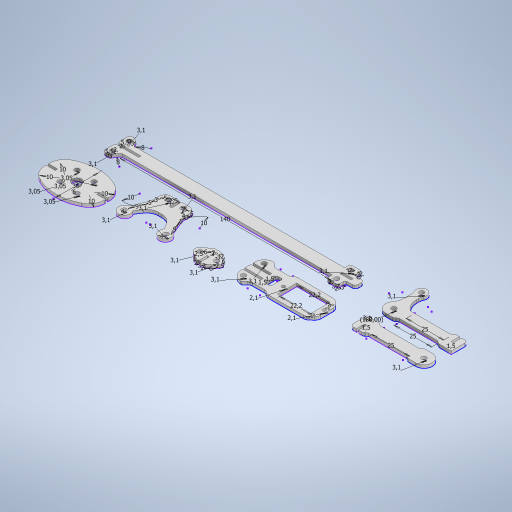
# Autodesk Inventor part: carbon_body_parts
Saved by Autodesk Inventor 2024 (Build 280153000, 153)
## iProperties
Created: 2024-04-09
Part Number: carbon_body_parts
Material: Generic
Document SubType Name: Modeling
Designer: nikop
Density: 1 g/cm^3
Appearance: Default
Author: nikop
Autodesk Inventor part; units mm, degrees
ref_plane "YZ Plane" through (0, 0, 0) normal (1, 0, 0) x (0, 1, 0)
ref_plane "XZ Plane" through (0, 0, 0) normal (0, 1, 0) x (-1, 0, 0)
ref_plane "XY Plane" through (0, 0, 0) normal (0, 0, 1) x (1, 0, 0)
sketch "Sketch1" plane through (0, 0, 0) normal (0, 1, 0) x (-1, 0, 0)
  circle A0 centre (58.9757, 25.2531) radius 1.525
  circle A1 centre (70.2894, 36.5668) radius 1.525
  circle A2 centre (57.915, 37.6275) radius 1.525
  circle A3 centre (71.3501, 24.1924) radius 1.525
  arc A4 (78.4011, 20.0636) -> (84.4011, 29.4099) centre (74.4027, 29.2295) ccw
  arc A5 (44.864, 29.4099) -> (50.864, 20.0636) centre (54.8624, 29.2295) ccw
  arc A6 (50.864, 20.0636) -> (78.4011, 20.0636) centre (64.6326, 46.7175) ccw
  arc A7 (84.4011, 32.4099) -> (78.4011, 41.7562) centre (74.4027, 32.5904) ccw
  arc A8 (50.864, 41.7562) -> (44.864, 32.4099) centre (54.8624, 32.5904) ccw
  arc A9 (78.4011, 41.7562) -> (50.864, 41.7562) centre (64.6326, 15.1024) ccw
  circle A10 centre (64.6326, 30.9099) radius 3
  line L0 (84.4011, 29.9099) -> (84.4011, 29.4099)
  line L1 (84.4011, 31.9099) -> (84.4011, 32.4099)
  line L2 (44.864, 29.9099) -> (44.864, 29.4099)
  line L3 (44.864, 31.9099) -> (44.864, 32.4099)
  line L4 (50.864, 31.6544) -> (50.864, 30.1544)
  line L5 (78.4011, 31.6599) -> (78.4011, 30.1599)
  line L6 (50.864, 30.1544) -> (50.864, 30.2794)
  line L7 (44.864, 29.9099) -> (44.864, 30.0349)
  line L8 (44.864, 31.7849) -> (44.864, 31.9099)
  line L9 (78.4011, 30.1599) -> (78.4011, 30.2849)
  line L10 (78.4011, 31.6599) -> (78.4011, 31.5349)
  line L11 (84.4011, 30.0349) -> (84.4011, 29.9099)
  line L12 (78.4011, 30.1599) -> (84.4011, 30.1599)
  line L13 (84.4011, 30.1599) -> (84.4011, 30.0349)
  line L14 (84.4011, 31.7849) -> (84.4011, 31.9099)
  line L15 (50.864, 30.1544) -> (44.864, 30.1544)
  line L16 (44.864, 30.1544) -> (44.864, 30.0349)
  line L17 (50.864, 31.6544) -> (44.864, 31.6544)
  line L18 (44.864, 31.6544) -> (44.864, 31.7849)
  line L19 (78.4011, 31.6599) -> (84.4011, 31.6599)
  line L20 (84.4011, 31.6599) -> (84.4011, 31.7849)
  line L21 (-81.7792, -0.1869) -> (-81.7792, -0.3869)
  arc A11 (-82.7792, -1.3869) -> (-81.7792, -0.3869) centre (-82.7792, -0.3869) ccw
  line L22 (-82.7792, -1.3869) -> (-86.2983, -1.3869)
  arc A12 (-86.2983, -1.3869) -> (-88.2983, -3.3869) centre (-86.2983, -3.3869) ccw
  line L23 (-88.2983, -3.3869) -> (-88.2983, -5.3869)
  arc A13 (-88.2983, -5.3869) -> (-86.2983, -7.3869) centre (-86.2983, -5.3869) ccw
  line L24 (-86.2983, -7.3869) -> (-82.7792, -7.3869)
  arc A14 (-81.7617, -8.3867) -> (-82.7792, -7.3869) centre (-82.7617, -8.3867) ccw
  line L25 (-81.7617, -8.3867) -> (-81.7617, -8.5869)
  line L26 (70.7017, -7.8869) -> (70.9617, -7.8869) construction
  line L27 (73.6839, -6.8202) -> (73.6839, -12.3202)
  arc A15 (71.1839, -13.3202) -> (73.6839, -12.3202) centre (71.4382, -10.331) ccw
  arc A16 (68.6839, -12.3202) -> (71.1839, -13.3202) centre (70.9296, -10.331) ccw
  line L28 (73.6995, -1.853) -> (73.6995, 3.647)
  arc A17 (73.6995, 3.647) -> (71.1995, 4.647) centre (71.4538, 1.6578) ccw
  arc A18 (71.1995, 4.647) -> (68.6839, 3.6292) centre (70.9452, 1.6578) ccw
  line L29 (-74.2088, -0.2378) -> (65.7912, -0.2378)
  line L30 (-74.2182, -8.5205) -> (65.7818, -8.5205)
  circle A19 centre (70.7017, 1.1131) radius 1.55
  circle A20 centre (70.7017, -9.8869) radius 1.55
  arc A21 (68.6839, -12.3202) -> (65.7818, -8.5205) centre (61.1656, -15.0543) ccw
  arc A22 (65.7912, -0.2378) -> (68.6839, 3.6292) centre (61.1303, 6.2643) ccw
  circle A23 centre (-77.7909, 0.3631) radius 1.55
  circle A24 centre (-77.7986, -9.1369) radius 1.55
  line L31 (-81.7617, -8.5869) -> (-81.7617, -11.5869)
  arc A25 (-81.7617, -11.5869) -> (-79.9139, -12.3522) centre (-80.175, -10.3693) ccw
  line L32 (-74.2182, -8.5205) -> (-74.2182, -11.5869)
  arc A26 (-76.0659, -12.3522) -> (-74.2182, -11.5869) centre (-75.8049, -10.3693) ccw
  line L33 (-79.9139, -12.3522) -> (-76.0659, -12.3522)
  line L34 (-81.7792, -0.1869) -> (-81.7792, 2.8131)
  line L35 (-74.2088, -0.2378) -> (-74.2088, 2.8131)
  arc A27 (-74.2088, 2.8131) -> (-76.0566, 3.5785) centre (-75.7955, 1.5956) ccw
  arc A28 (-79.9314, 3.5785) -> (-81.7792, 2.8131) centre (-80.1925, 1.5956) ccw
  line L36 (-79.9314, 3.5785) -> (-76.0566, 3.5785)
  line L37 (58.2017, -5.1369) -> (72.9149, -5.1369)
  line L38 (58.2017, -3.6369) -> (72.9149, -3.6369)
  line L39 (58.2017, -3.6369) -> (58.2017, -5.1369)
  arc A29 (72.9149, -3.6369) -> (73.6995, -1.853) centre (71.7084, -2.0417) ccw
  arc A30 (73.6839, -6.8202) -> (72.9149, -5.1369) centre (71.6866, -6.7153) ccw
  line L40 (-83.2983, -5.1369) -> (-75.7983, -5.1369)
  line L41 (-83.2983, -3.6369) -> (-75.7983, -3.6369)
  line L42 (-75.7983, -3.6369) -> (-75.7983, -5.1369)
  line L43 (-83.2983, -3.6369) -> (-83.2983, -5.1369)
  line L44 (-23.6125, 23.696) -> (-22.1233, 23.696)
  line L45 (-22.1233, 23.696) -> (-20.6203, 23.6923)
  arc A31 (-18.7385, 36.0083) -> (-20.6179, 36.6923) centre (-20.6455, 33.6924) ccw
  arc A32 (-20.6203, 23.6923) -> (-18.7409, 24.3763) centre (-20.648, 26.6922) ccw
  arc A33 (-23.634, 36.696) -> (-25.5134, 36.012) centre (-23.6063, 33.6962) ccw
  arc A34 (-25.4919, 24.3801) -> (-23.6125, 23.696) centre (-23.5848, 26.6959) ccw
  circle A35 centre (-27.6234, 30.215) radius 1.55
  circle A36 centre (-16.6231, 30.2237) radius 1.55
  line L46 (-25.5134, 36.012) -> (-30.1097, 32.1553)
  line L47 (-25.4919, 24.3801) -> (-30.0881, 28.2368)
  arc A37 (-30.1097, 32.1553) -> (-30.0881, 28.2368) centre (-28.5461, 30.2046) ccw
  line L48 (-18.7409, 24.3763) -> (-14.1446, 28.2331)
  line L49 (-18.7385, 36.0083) -> (-14.1422, 32.1515)
  arc A38 (-14.1446, 28.2331) -> (-14.1422, 32.1515) centre (-15.6963, 30.1933) ccw
  line L50 (-23.634, 36.696) -> (-23.1232, 36.696)
  line L51 (-21.1071, 36.6935) -> (-20.6179, 36.6923)
  line L52 (-22.8732, 30.1867) -> (-22.8732, 36.696)
  line L53 (-22.8732, 36.696) -> (-23.1232, 36.696)
  line L54 (-21.3733, 30.1867) -> (-21.3733, 36.6935)
  line L55 (-21.3733, 36.6935) -> (-21.1071, 36.6935)
  line L56 (-22.8732, 30.1867) -> (-21.3733, 30.1867)
  arc A39 (-117.1771, -18.2977) -> (-116.557, -15.6154) centre (-122.5569, -15.641) ccw
  arc A40 (-117.1771, -18.2977) -> (-110.9285, -18.2954) centre (-114.0522, -19.8741) ccw
  arc A41 (-111.557, -15.622) -> (-110.9285, -18.2954) centre (-105.557, -15.622) ccw
  arc A42 (-109.6182, -4.6979) -> (-111.557, -10.5979) centre (-101.6102, -10.5979) ccw
  arc A43 (-109.6182, -4.6979) -> (-114.0537, 4.0542) centre (-114.0537, -1.4458) ccw
  line L57 (-114.0537, 4.0542) -> (-118.7253, 4.0542)
  arc A44 (-118.7253, 4.0542) -> (-120.1395, 3.4684) centre (-118.7253, 2.0542) ccw
  line L58 (-120.1395, 3.4684) -> (-120.4679, 3.14)
  arc A45 (-121.8822, 2.5542) -> (-120.4679, 3.14) centre (-121.8822, 4.5542) ccw
  line L59 (-146.8822, 2.5542) -> (-148.5338, 3.5078)
  arc A46 (-148.5338, 3.5078) -> (-149.9966, 4.0093) centre (-149.8634, 2.0137) ccw
  line L60 (-149.9966, 4.0093) -> (-155.6682, 4.0093)
  arc A47 (-149.9966, -6.9907) -> (-148.5824, -6.4049) centre (-149.9966, -4.9907) ccw
  line L61 (-148.5824, -6.4049) -> (-148.254, -6.0765)
  arc A48 (-146.8822, -5.4458) -> (-148.254, -6.0765) centre (-146.7944, -7.4439) ccw
  arc A49 (-120.4679, -6.0316) -> (-121.8822, -5.4458) centre (-121.8822, -7.4458) ccw
  line L62 (-120.4679, -6.0316) -> (-119.4827, -7.0169)
  arc A50 (-116.557, -14.0847) -> (-119.4827, -7.0169) centre (-126.557, -14.0847) ccw
  arc A51 (-146.2322, 21.7443) -> (-144.8179, 21.1585) centre (-144.8179, 23.1585) ccw
  line L63 (-146.2322, 21.7443) -> (-146.5606, 22.0727)
  arc A52 (-146.5606, 22.0727) -> (-147.9748, 22.6585) centre (-147.9748, 20.6585) ccw
  line L64 (-147.9748, 22.6585) -> (-152.6464, 22.6585)
  arc A53 (-152.6464, 22.6585) -> (-158.1464, 17.1585) centre (-152.6464, 17.1585) ccw
  arc A54 (-158.1464, 17.1585) -> (-152.6464, 11.6585) centre (-152.6464, 17.1585) ccw
  line L65 (-152.6464, 11.6585) -> (-147.9748, 11.6585)
  arc A55 (-147.9748, 11.6585) -> (-146.5606, 12.2443) centre (-147.9748, 13.6585) ccw
  line L66 (-146.5606, 12.2443) -> (-146.2322, 12.5727)
  arc A56 (-144.8179, 13.1585) -> (-146.2322, 12.5727) centre (-144.8179, 11.1585) ccw
  arc A57 (-118.6935, 12.6308) -> (-119.8179, 13.1585) centre (-120.0634, 11.1736) ccw
  line L67 (-118.6935, 12.6308) -> (-118.3651, 12.3024)
  arc A58 (-118.3651, 12.3024) -> (-116.9509, 11.7166) centre (-116.9509, 13.7166) ccw
  line L68 (-116.9509, 11.7166) -> (-111.2793, 11.7166)
  arc A59 (-116.9509, 22.7166) -> (-118.3651, 22.1308) centre (-116.9509, 20.7166) ccw
  line L69 (-118.3651, 22.1308) -> (-118.6935, 21.8024)
  arc A60 (-119.8179, 21.1585) -> (-118.6935, 21.8024) centre (-120.196, 23.1224) ccw
  line L70 (-157.6682, -1.4907) -> (-157.6682, -4.9907)
  line L71 (-157.6682, -1.4907) -> (-157.6682, 2.0093)
  arc A61 (-157.6682, -4.9907) -> (-155.6682, -6.9907) centre (-155.6682, -4.9907) ccw
  line L72 (-109.2793, 17.2166) -> (-109.2793, 20.7166)
  line L73 (-109.2793, 17.2166) -> (-109.2793, 13.7166)
  arc A62 (-109.2793, 20.7166) -> (-111.2793, 22.7166) centre (-111.2793, 20.7166) ccw
  line L74 (-149.9966, -6.9907) -> (-151.1682, -6.9907)
  line L75 (-154.1651, -6.9907) -> (-155.6682, -6.9907)
  circle A63 centre (-114.0537, -1.4458) radius 1.55
  circle A64 centre (-114.0602, -19.8581) radius 1.55
  circle A65 centre (-152.6464, 17.1585) radius 1.55
  line L76 (-111.2793, 22.7166) -> (-112.7793, 22.7166)
  line L77 (-115.7793, 22.7166) -> (-116.9509, 22.7166)
  line L78 (-111.557, -15.622) -> (-111.557, -10.5979)
  line L79 (-116.557, -15.6154) -> (-116.557, -14.0847)
  line L80 (-121.8822, -5.4458) -> (-146.8822, -5.4458)
  line L81 (-121.8822, 2.5542) -> (-146.8822, 2.5542)
  line L82 (-144.8179, 13.1585) -> (-119.8179, 13.1585)
  line L83 (-144.8179, 21.1585) -> (-119.8179, 21.1585)
  line L84 (-155.6682, 4.0093) -> (-157.6682, 4.0093)
  line L85 (-157.6682, 4.0093) -> (-157.6682, 2.0093)
  line L86 (-111.2793, 11.7166) -> (-109.2793, 11.7166)
  line L87 (-111.2793, 11.7166) -> (-113.2793, 11.7166) construction
  line L88 (-109.2793, 11.7166) -> (-109.2793, 13.7166)
  line L89 (-151.2682, -6.9907) -> (-151.1682, -6.9907)
  line L90 (-154.0682, -6.9907) -> (-154.1651, -6.9907)
  line L91 (-115.6793, 22.7166) -> (-115.7793, 22.7166)
  line L92 (-112.8793, 22.7166) -> (-112.7793, 22.7166)
  line L93 (-151.6682, -6.9907) -> (-151.2682, -6.9907)
  line L94 (-153.6682, -1.4907) -> (-153.6682, -6.9907)
  line L95 (-153.6682, -6.9907) -> (-154.0682, -6.9907)
  line L96 (-113.2793, 17.2166) -> (-113.2793, 22.7166)
  line L97 (-113.2793, 22.7166) -> (-112.8793, 22.7166)
  line L98 (-115.2793, 22.7166) -> (-115.6793, 22.7166)
  line L99 (-113.2793, 17.2166) -> (-114.7793, 17.2166)
  line L100 (-114.7793, 17.2166) -> (-114.7793, 22.7166)
  line L101 (-114.7793, 22.7166) -> (-115.2793, 22.7166)
  line L102 (-153.6682, -1.4907) -> (-152.1682, -1.4907)
  line L103 (-152.1682, -1.4907) -> (-152.1682, -6.9907)
  line L104 (-152.1682, -6.9907) -> (-151.6682, -6.9907)
  line L105 (-47.726, 11.8652) -> (-47.014, 11.8652)
  arc A66 (-47.014, 11.8652) -> (-41.014, 17.8652) centre (-47.014, 17.8652) ccw
  arc A67 (-41.014, 27.5152) -> (-47.014, 33.5152) centre (-47.014, 27.5152) ccw
  line L106 (-47.014, 33.5152) -> (-47.726, 33.5152)
  line L107 (-89.264, 28.1152) -> (-89.264, 22.6902)
  line L108 (-89.264, 22.6902) -> (-89.264, 17.2652)
  line L109 (-47.726, 11.8652) -> (-49.6723, 13.8116)
  line L110 (-87.6912, 12.8652) -> (-64.2306, 12.8652)
  line L111 (-62.1093, 13.7439) -> (-62.0417, 13.8116)
  line L112 (-53.226, 14.6902) -> (-51.7936, 14.6902)
  line L113 (-53.226, 14.6902) -> (-59.9203, 14.6902)
  line L114 (-93.564, 22.6902) -> (-93.564, 18.6074)
  line L115 (-92.2884, 15.6787) -> (-90.4156, 13.9365)
  arc A68 (-93.564, 18.6074) -> (-92.2884, 15.6787) centre (-89.564, 18.6074) ccw
  arc A69 (-90.4156, 13.9365) -> (-87.6912, 12.8652) centre (-87.6912, 16.8652) ccw
  arc A70 (-49.6723, 13.8116) -> (-51.7936, 14.6902) centre (-51.7936, 11.6902) ccw
  arc A71 (-59.9203, 14.6902) -> (-62.0417, 13.8116) centre (-59.9203, 11.6902) ccw
  arc A72 (-64.2306, 12.8652) -> (-62.1093, 13.7439) centre (-64.2306, 15.8652) ccw
  line L116 (-47.726, 33.5152) -> (-49.6723, 31.5689)
  line L117 (-87.6912, 32.5152) -> (-64.2306, 32.5152)
  line L118 (-62.1093, 31.6366) -> (-62.0417, 31.5689)
  line L119 (-53.226, 30.6902) -> (-51.7936, 30.6902)
  line L120 (-53.226, 30.6902) -> (-59.9203, 30.6902)
  line L121 (-93.564, 22.6902) -> (-93.564, 26.7731)
  line L122 (-92.2884, 29.7018) -> (-90.4156, 31.444)
  arc A73 (-92.2884, 29.7018) -> (-93.564, 26.7731) centre (-89.564, 26.7731) ccw
  arc A74 (-87.6912, 32.5152) -> (-90.4156, 31.444) centre (-87.6912, 28.5152) ccw
  arc A75 (-51.7936, 30.6902) -> (-49.6723, 31.5689) centre (-51.7936, 33.6902) ccw
  arc A76 (-62.0417, 31.5689) -> (-59.9203, 30.6902) centre (-59.9203, 33.6902) ccw
  arc A77 (-62.1093, 31.6366) -> (-64.2306, 32.5152) centre (-64.2306, 29.5152) ccw
  line L123 (-57.226, 18.6902) -> (-59.164, 18.6902)
  line L124 (-60.164, 19.6902) -> (-60.164, 25.6902)
  line L125 (-56.226, 19.6902) -> (-56.226, 25.6902)
  line L126 (-57.226, 26.6902) -> (-59.164, 26.6902)
  arc A78 (-57.226, 18.6902) -> (-56.226, 19.6902) centre (-57.226, 19.6902) ccw
  arc A79 (-60.164, 19.6902) -> (-59.164, 18.6902) centre (-59.164, 19.6902) ccw
  arc A80 (-59.164, 26.6902) -> (-60.164, 25.6902) centre (-59.164, 25.6902) ccw
  arc A81 (-56.226, 25.6902) -> (-57.226, 26.6902) centre (-57.226, 25.6902) ccw
  line L127 (-41.014, 17.8652) -> (-41.014, 18.1902)
  line L128 (-89.264, 17.2652) -> (-89.264, 16.2652)
  line L129 (-89.264, 28.1152) -> (-89.264, 29.1152)
  line L130 (-89.264, 16.2652) -> (-67.064, 16.2652)
  line L131 (-89.264, 29.1152) -> (-67.064, 29.1152)
  line L132 (-67.064, 16.2652) -> (-67.064, 29.1152)
  line L133 (-41.014, 27.5152) -> (-41.014, 27.1902)
  line L134 (-41.014, 21.1902) -> (-41.014, 24.1902)
  circle A82 centre (-44.926, 29.5902) radius 1.55
  circle A83 centre (-44.926, 15.7902) radius 1.55
  circle A84 centre (-64.614, 22.6902) radius 1.05
  circle A85 centre (-91.714, 22.6902) radius 1.05
  line L135 (-41.014, 18.6902) -> (-41.014, 18.1902)
  line L136 (-53.226, 20.6902) -> (-41.014, 20.6902)
  line L137 (-41.014, 20.6902) -> (-41.014, 21.1902)
  line L138 (-53.226, 24.6902) -> (-41.014, 24.6902)
  line L139 (-41.014, 24.6902) -> (-41.014, 24.1902)
  line L140 (-41.014, 26.6902) -> (-41.014, 27.1902)
  line L141 (-53.226, 24.6902) -> (-53.226, 26.1902)
  line L142 (-53.226, 26.1902) -> (-41.014, 26.1902)
  line L143 (-41.014, 26.1902) -> (-41.014, 26.6902)
  line L144 (-53.226, 20.6902) -> (-53.226, 19.1902)
  line L145 (-53.226, 19.1902) -> (-41.014, 19.1902)
  line L146 (-41.014, 19.1902) -> (-41.014, 18.6902)
  line L147 (10.9194, 25.0056) -> (8.2063, 29.0278)
  line L148 (26.5678, 25.0056) -> (29.2808, 29.0278)
  line L149 (18.7436, 21.4792) -> (17.5517, 21.4792)
  line L150 (18.7436, 21.4792) -> (19.9355, 21.4792)
  arc A86 (10.9194, 25.0056) -> (17.5517, 21.4792) centre (17.5517, 29.4792) ccw
  arc A87 (19.9355, 21.4792) -> (26.5678, 25.0056) centre (19.9355, 29.4792) ccw
  circle A88 centre (4.7436, 31.4792) radius 1.55
  circle A89 centre (32.7436, 31.4792) radius 1.55
  circle A90 centre (13.9936, 10.9792) radius 1.55
  circle A91 centre (23.4936, 10.9792) radius 1.55
  line L151 (17.2436, 7.9792) -> (12.2436, 7.9792)
  arc A92 (8.708, 11.5147) -> (12.2436, 7.9792) centre (12.6837, 11.9549) ccw
  line L152 (8.708, 11.5147) -> (8.708, 14.5147)
  arc A93 (8.708, 14.5147) -> (7.7326, 19.4186) centre (-1.2761, 15.0777) ccw
  line L153 (7.7326, 19.4186) -> (4.2884, 27.7336)
  arc A94 (8.2063, 29.0278) -> (4.2884, 27.7336) centre (5.1725, 31.6347) ccw
  line L154 (17.7436, 7.9792) -> (17.2436, 7.9792)
  line L155 (19.7436, 7.9792) -> (20.2436, 7.9792)
  line L156 (20.2436, 7.9792) -> (25.2436, 7.9792)
  arc A95 (25.2436, 7.9792) -> (28.7791, 11.5147) centre (24.8034, 11.9549) ccw
  line L157 (28.7791, 11.5147) -> (28.7791, 14.5147)
  arc A96 (29.7545, 19.4186) -> (28.7791, 14.5147) centre (38.7632, 15.0777) ccw
  line L158 (29.7545, 19.4186) -> (33.1987, 27.7336)
  arc A97 (33.1987, 27.7336) -> (29.2808, 29.0278) centre (32.3147, 31.6347) ccw
  line L159 (19.4936, 14.4792) -> (19.4936, 7.9792)
  line L160 (19.4936, 7.9792) -> (19.7436, 7.9792)
  line L161 (17.9936, 14.4792) -> (17.9936, 7.9792)
  line L162 (17.9936, 7.9792) -> (17.7436, 7.9792)
  line L163 (17.9936, 14.4792) -> (19.4936, 14.4792)
  point P0 (-118.6935, 21.8024)
  point P1 (-152.6464, 11.6585)
  point P2 (-146.5606, 12.2443)
  point P3 (-116.9509, 11.7166)
  point P4 (-120.1395, 3.4684)
  point P5 (-149.9966, 4.0093)
  point P6 (-148.5824, -6.4049)
  point P7 (-47.014, 33.5152)
  point P8 (-87.6912, 32.5152)
  point P9 (-93.564, 26.7731)
  point P10 (-64.2306, 12.8652)
  point P11 (-59.164, 18.6902)
  point P12 (-60.164, 19.6902)
  point P13 (-57.226, 26.6902)
  point P14 (-56.226, 25.6902)
  point P15 (-56.226, 19.6902)
  point P16 (-88.2983, -5.3869)
  point P17 (-82.7792, -7.3869)
  point P18 (8.708, 11.5147)
  dimension "d150" = 3.05
  dimension "d151" = 3.05
  dimension "d152" = 3.05
  dimension "d153" = 3.05
  dimension "d154" = 10
  dimension "d155" = 10
  dimension "d156" = 30
  dimension "d157" = 10
  dimension "d158" = 10
  dimension "d159" = 30
  dimension "d160" = 6
  dimension "d183" = 5.5
  dimension "d184" = 3
  dimension "d185" = 3
  dimension "d186" = 5.5
  dimension "d187" = 3
  dimension "d188" = 3
  dimension "d189" = 140
  dimension "d191" = 3.1
  dimension "d192" = 3.1
  dimension "d193" = 8
  dimension "d194" = 8
  dimension "d195" = 3.1
  dimension "d196" = 3
  dimension "d197" = 2
  dimension "d198" = 2
  dimension "d199" = 2
  dimension "d200" = 2
  dimension "d201" = 3
  dimension "d202" = 2
  dimension "d203" = 2
  dimension "d204" = 2
  dimension "d205" = 2
  dimension "d220" = 2
  dimension "d221" = 2
  dimension "d222" = 2
  dimension "d223" = 3
  dimension "d224" = 2
  dimension "d225" = 3
  dimension "d226" = 2
  dimension "d227" = 3
  dimension "d228" = 2
  dimension "d229" = 3
  dimension "d230" = 3.1
  dimension "d231" = 3.1
  dimension "d232" = 6
  dimension "d233" = 6
  dimension "d234" = 2.5
  dimension "d235" = 6
  dimension "d236" = 6
  dimension "d237" = 2.5
  dimension "d238" = 3.1
  dimension "d239" = 3.1
  dimension "d240" = 3.1
  dimension "d241" = 25
  dimension "d242" = 25
  dimension "d243" = 25
  dimension "d244" = 2
  dimension "d245" = 180
  dimension "d246" = 1.5
  dimension "d247" = 1.5
  dimension "d248" = 1
  dimension "d249" = 1
  dimension "d250" = 22.2
  constraints: 328 end point, 153 point on circle, 98 centre point, 22 perpendicular, 16 vertical, 14 horizontal, 7 point on line, 4 collinear, 2 parallel, 1 tangent
  measures "d150" diameter of A0
  measures "d151" diameter of A1
  measures "d152" diameter of A2
  measures "d153" diameter of A3
  measures "d154" radius of A4
  measures "d155" radius of A5
  measures "d156" radius of A6
  measures "d157" radius of A7
  measures "d158" radius of A8
  measures "d159" radius of A9
  measures "d160" diameter of A10
  measures "d183" distance of L27.start L27.end
  measures "d184" radius of A15
  measures "d185" radius of A16
  measures "d186" distance of L28.start L28.end
  measures "d187" radius of A17
  measures "d188" radius of A18
  measures "d189" distance of L29.start L29.end
  measures "d191" diameter of A19
  measures "d192" diameter of A20
  measures "d193" radius of A21
  measures "d194" radius of A22
  measures "d195" diameter of A24
  measures "d196" distance of L31.start L31.end
  measures "d197" distance of L31.end L33.start
  measures "d198" radius of A25
  measures "d199" distance of L32.end L33.end
  measures "d200" radius of A26
  measures "d201" distance of L21.start L34.end
  measures "d202" distance of L35.end L36.end
  measures "d203" radius of A27
  measures "d204" distance of L34.end L36.start
  measures "d205" radius of A28
  measures "d220" radius of A29
  measures "d221" radius of A30
  measures "d222" distance of L51.end L49.start
  measures "d223" radius of A31
  measures "d224" distance of L45.end L48.start
  measures "d225" radius of A32
  measures "d226" distance of L50.start L46.start
  measures "d227" radius of A33
  measures "d228" distance of L44.start L47.start
  measures "d229" radius of A34
  measures "d230" diameter of A35
  measures "d231" diameter of A36
  measures "d232" distance of L46.start L46.end
  measures "d233" distance of L47.start L47.end
  measures "d234" radius of A37
  measures "d235" distance of L48.start L48.end
  measures "d236" distance of L49.start L49.end
  measures "d237" radius of A38
  measures "d238" diameter of A63
  measures "d239" diameter of A64
  measures "d240" diameter of A65
  measures "d241" distance of L80.start L80.end
  measures "d242" distance of L81.start L59.start
  measures "d243" distance of L83.start L83.end
  measures "d244" distance of L86.start L88.start
  measures "d245" angle of L86 L87
  measures "d246" distance of L99.start L99.end
  measures "d247" distance of L102.start L102.end
  measures "d248" distance of L108.end L130.start
  measures "d249" distance of L107.start L129.end
  measures "d250" distance of L130.start L132.start
extrude "Extrusion1" add sketch "Sketch1" along normal blind 2
body "Solid1"
